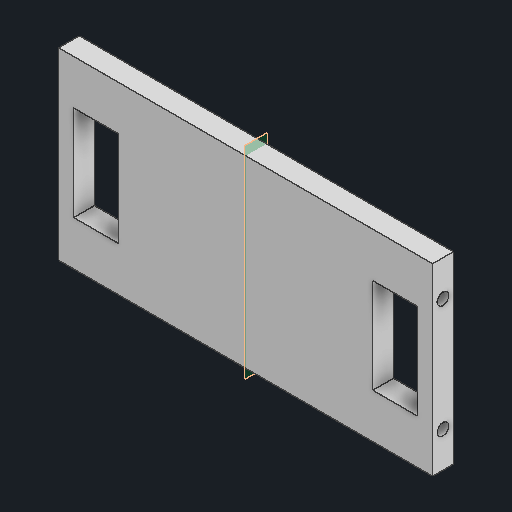
# Autodesk Inventor part: base3
Saved by Autodesk Inventor 2026 (Build 300175000, 175)
## iProperties
Created: 2026-08-17
Part Number: base3
Material: Generic
Document SubType Name: Modeling
Designer: imcle
Density: 1 g/cm^3
Appearance: Default
Author: imcle
Autodesk Inventor part; units mm, degrees
ref_plane "YZ Plane" through (0, 0, 0) normal (1, 0, 0) x (0, 1, 0)
ref_plane "XZ Plane" through (0, 0, 0) normal (0, 1, 0) x (-1, 0, 0)
sketch "Sketch2" plane through (0, 0, 0) normal (0, 0, 1) x (1, 0, 0)
  line L0 (0, 0) -> (126, 0)
  line L1 (126, 0) -> (126, 60)
  line L2 (126, 60) -> (0, 60)
  line L3 (0, 60) -> (0, 0)
  dimension "d1" = 126
  dimension "d2" = 60
  constraints: 8 end point, 2 parallel, 1 horizontal, 1 perpendicular
  measures "d1" distance of L2.end L1.end
  measures "d2" distance of L1.end L0.end
extrude "Extrusion1" add sketch "Sketch2" along normal blind 7
sketch "Sketch3" plane through (126, 0, 0) normal (1, 0, 0) x (0, 0, -1)
  line L0 (0, 0) -> (-7, 0) projected
  line L1 (-3.5, 0) -> (-3.5, 11)
  circle A0 centre (-3.5, 11) radius 2
  dimension "d5" = 11
  dimension "d6" = 4
  constraints: 2 end point, 1 centre point, 1 coincident, 1 midpoint, 1 vertical
  measures "d5" distance of L1.start L1.end
  measures "d6" diameter of A0
extrude "Extrusion2" cut sketch "Sketch3" against normal blind 5.5
pattern_linear "Rectangular Pattern1" count 2 spacing -120.5 along (1, 0, 0) count 2 spacing 38 along (0, 1, 0) of "Extrusion2"
sketch "Sketch4" plane through (0, 0, 0) normal (0, -1, 0) x (1, 0, 0)
  line L0 (0, 7) -> (126, 7) projected
  line L1 (0, 0) -> (126, 0)
  line L2 (126, 0) -> (126, 7)
  line L3 (126, 7) -> (0, 7)
  line L4 (0, 7) -> (0, 0)
  constraints: 8 end point, 2 parallel, 1 horizontal, 1 perpendicular
ref_plane "Work Plane1" through (0, 30, 0) normal (0, -1, 0) x (1, 0, 0)
extrude "Extrusion3" add sketch "Sketch4" along normal blind 1
mirror "Mirror1" about plane through (0, 30, 0) normal (0, -1, 0) of "Extrusion3"
sketch "Sketch5" plane through (0, 0, 0) normal (0, 0, -1) x (-1, 0, 0)
  line L0 (0, 61) -> (-126, 61) projected
  line L1 (0, -1) -> (0, 61) projected
  line L2 (0, 30) -> (-63, 30)
  line L3 (-63, 50) -> (-63, 10)
  circle A0 centre (-63, 10) radius 2
  circle A1 centre (-63, 50) radius 2
  point P0 (0, 0)
  dimension "d17" = 40
  dimension "d18" = 4
  constraints: 4 end point, 2 centre point, 2 midpoint, 1 coincident, 1 horizontal, 1 symmetric about line, 1 vertical, 1 other
  measures "d17" distance of L3.start L3.end
  measures "d18" diameter of A0
extrude "Extrusion4" cut sketch "Sketch5" against normal blind 5.5
sketch "Sketch7" plane through (0, 0, 0) normal (0, 0, -1) x (-1, 0, 0)
  line L0 (0, -1) -> (0, 61) projected
  line L1 (0, 30) -> (-25.15, 30)
  line L2 (0, 30) -> (-5, 30)
  line L3 (-25.15, 30) -> (-20.15, 30)
  line L4 (-12.575, -1) -> (-12.575, 14)
  line L5 (-12.575, -1) -> (2.425, -1) construction
  line L6 (-5.075, 14) -> (-20.15, 14)
  line L7 (-20.15, 14) -> (-20.15, 46)
  line L8 (-20.15, 46) -> (-5.075, 46)
  line L9 (-5.075, 46) -> (-5.075, 14)
  point P0 (0, 0)
  dimension "d29" = 25.15
  dimension "d30" = 5
  dimension "d31" = 5
  dimension "d32" = 15
  dimension "d33" = 90
  dimension "d34" = 32
  constraints: 18 end point, 3 horizontal, 2 parallel, 2 perpendicular, 2 point on line, 1 midpoint, 1 vertical
  measures "d29" distance of L1.start L1.end
  measures "d30" distance of L1.start L2.end
  measures "d31" distance of L1.end L3.end
  measures "d32" distance of L4.start L4.end
  measures "d33" angle of L5 L4
  measures "d34" distance of L6.end L7.end
extrude "Extrusion6" cut sketch "Sketch7" against normal up to surface (7 mm away)
ref_plane "Work Plane2" through (63, -1, 0) normal (-1, 0, 0) x (0, 0, 1)
mirror "Mirror2" about plane through (63, -1, 0) normal (-1, 0, 0) of "Extrusion6"
body "Solid2"
